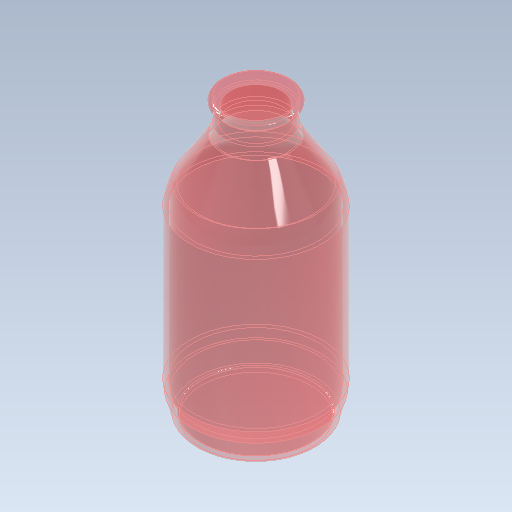
# Autodesk Inventor part: 100ml Bottle 2
Saved by Autodesk Inventor 2021 (Build 250183000, 183)
## iProperties
Created: 2019-11-05
Part Number: 100ml Bottle 2
Material: Glass
Document SubType Name: Modeling
Designer: jgray
Density: 2.18 g/cm^3
Appearance: Dark Red
Author: jgray
Autodesk Inventor part; units mm, degrees
ref_plane "YZ Plane" through (0, 0, 0) normal (1, 0, 0) x (0, 1, 0)
ref_plane "XZ Plane" through (0, 0, 0) normal (0, 1, 0) x (-1, 0, 0)
ref_plane "XY Plane" through (0, 0, 0) normal (0, 0, 1) x (1, 0, 0)
sketch "Sketch1" plane through (0, 0, 0) normal (0, 1, 0) x (-1, 0, 0)
  circle A0 centre (0, 0) radius 23.75
  dimension "d0" = 47.5
  constraints: 1 centre point, 1 coincident
  measures "d0" diameter of A0
extrude "Extrusion1" add sketch "Sketch1" along normal blind 90
chamfer "Chamfer1" distance 10 angle 15 1 edges at (23.75, 0, 0) measured on face at (-23.673, 60, -1.9111)
chamfer "Chamfer2" distance 12.5 distance2 20 1 edges at (23.75, 90, 0) measured on face at (-5.9257, 90, 5.2497)
sketch "Sketch2" plane through (0, 90, 0) normal (0, 1, 0) x (1, 0, 0)
  circle A0 centre (0, 0) radius 11.25 projected
  circle A1 centre (0, 0) radius 11.25
  constraints: 1 centre point, 1 coincident, 1 concentric
extrude "Extrusion2" add sketch "Sketch2" along normal blind 7 draft -5
fillet "Fillet6" radius 2 1 edges at (21.0705, 0, 0)
fillet "Fillet5" radius 15 1 edges at (23.75, 10, 0)
fillet "Fillet4" radius 15 1 edges at (23.75, 70, 0)
fillet "Fillet3" radius 8 2 edges at (0, 90, -11.25) (0, 90, 11.25)
shell "Shell1" thickness 1.5 removed faces 1 at (1.8241, 97, -2.1468)
sketch "Sketch3" plane through (0, 97, 0) normal (0, 1, 0) x (1, 0, 0)
  circle A0 centre (0, 0) radius 12.5
  dimension "d11" = 25
  constraints: 1 centre point, 1 coincident
  measures "d11" diameter of A0
extrude "Extrusion3" add sketch "Sketch3" along normal blind 3
fillet "Fillet1" radius 1.5 2 edges at (-12.5, 100, 0) (-12.5, 97, 0)
fillet "Fillet2" radius 0.5 1 edges at (-10.6376, 97, 0)
body "Solid1"
